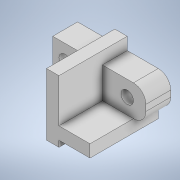
# Autodesk Inventor part: oled_support
Saved by Autodesk Inventor 2021 (Build 250183000, 183)
## iProperties
Created: 2024-12-22
Part Number: oled_support
Material: Generic
Document SubType Name: Modeling
Designer: Toby
Density: 1 g/cm^3
Appearance: Default
Author: Toby
Autodesk Inventor part; units mm, degrees
ref_plane "YZ Plane" through (0, 0, 0) normal (1, 0, 0) x (0, 1, 0)
ref_plane "XZ Plane" through (0, 0, 0) normal (0, 1, 0) x (-1, 0, 0)
ref_plane "XY Plane" through (0, 0, 0) normal (0, 0, 1) x (1, 0, 0)
sketch "Sketch1" plane through (0, 0, 0) normal (0, 0, 1) x (1, 0, 0)
  line L0 (-6.2132, 2.886) -> (8.7868, 2.886)
  line L1 (8.7868, 2.886) -> (8.7868, -2.114)
  line L2 (8.7868, -2.114) -> (-6.2132, -2.114)
  line L3 (-6.2132, -2.114) -> (-6.2132, 2.886)
  point P0 (0, 0)
  dimension "d0" = 15
  dimension "d1" = 5
  constraints: 8 end point, 2 parallel, 1 horizontal, 1 perpendicular
  measures "d0" distance of L0.start L0.end
  measures "d1" distance of L2.end L0.start
extrude "Extrusion1" add sketch "Sketch1" along normal blind 4
sketch "Sketch2" plane through (0, 0, 0) normal (0, 0, -1) x (-1, 0, 0)
  line L0 (-8.7868, 2.886) -> (6.2132, 2.886) projected
  line L1 (6.2132, 2.886) -> (6.2132, -2.114) projected
  point P0 (0, 0)
  point P1 (4.2132, 0.386)
  point P2 (-5.7868, 0.386)
  dimension "d4" = 2.5
  dimension "d5" = 2.5
  dimension "d6" = 2
  dimension "d7" = 10
  measures "d4" distance from line of L0 point (4.213, 0.386)
  measures "d5" distance from line of L0 point (-5.787, 0.386)
  measures "d6" distance from line of L1 point (4.213, 0.386)
  measures "d7" distance of point (4.213, 0.386) point (-5.787, 0.386)
hole "Hole1" at (-4.2132, 0.386, 0) at (5.7868, 0.386, 0) direction (0, 0, 1) diameter 2 depth 4 tip angle 118
sketch "Sketch3" plane through (0, 0, 0) normal (0, 0, -1) x (-1, 0, 0)
  line L0 (-8.7868, 2.886) -> (6.2132, 2.886) projected
  line L1 (0.2132, 2.886) -> (-1.7868, 2.886)
  line L2 (-1.7868, 2.886) -> (-1.7868, -7.114)
  line L3 (-1.7868, -7.114) -> (0.2132, -7.114)
  line L4 (0.2132, -7.114) -> (0.2132, 2.886)
  line L5 (6.2132, 2.886) -> (6.2132, -2.114) projected
  line L6 (-1.7868, 2.886) -> (0.2132, 2.886)
  line L7 (0.2132, 2.886) -> (0.2132, 4.886)
  line L8 (0.2132, 4.886) -> (-1.7868, 4.886)
  line L9 (-1.7868, 4.886) -> (-1.7868, 2.886)
  point P0 (0, 0)
  dimension "d15" = 6
  dimension "d16" = 2
  dimension "d17" = 12
  dimension "d18" = 2
  constraints: 16 end point, 4 parallel, 2 horizontal, 2 perpendicular, 1 collinear, 1 point on line
  measures "d15" distance between parallel lines of L5 L4
  measures "d16" distance of L2.end L3.end
  measures "d17" distance between parallel lines of L3 L8
  measures "d18" distance between parallel lines of L0 L8
extrude "Extrusion2" add sketch "Sketch3" against normal blind 11
fillet "Fillet1" radius 2 2 edges at (8.7868, 2.886, 2) (8.7868, -2.114, 2)
sketch "Sketch4" plane through (1.7868, -2.114, 0) normal (0, -1, 0) x (1, 0, 0)
  line L0 (0, 0) -> (0, 11) projected
  line L1 (7, 0) -> (5, 0) projected
  line L2 (0, 11) -> (5, 11)
  line L3 (5, 11) -> (5, 0)
  line L4 (5, 0) -> (0, 0)
  line L5 (0, 0) -> (0, 11)
  point P0 (-1.7868, 0)
  constraints: 8 end point, 2 parallel, 1 horizontal, 1 perpendicular
extrude "Extrusion3" add sketch "Sketch4" along normal blind 2
sketch "Sketch5" plane through (-0.2132, -7.114, 0) normal (0, -1, 0) x (1, 0, 0)
  line L0 (-6, 0) -> (-6, 4) projected
  line L1 (7, 11) -> (2, 11) projected
  line L2 (-6, 0) -> (7, 0)
  line L3 (7, 0) -> (7, 11)
  line L4 (7, 11) -> (-6, 11)
  line L5 (-6, 11) -> (-6, 0)
  point P0 (0.2132, 0)
  point P1 (2, 11)
  constraints: 8 end point, 2 parallel, 1 horizontal, 1 perpendicular
extrude "Extrusion4" cut sketch "Sketch5" against normal blind 2
body "Solid1"
